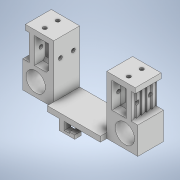
# Autodesk Inventor part: suporte estruzor 1
Saved by Autodesk Inventor 2022 (Build 260153000, 153)
## iProperties
Created: 2022-02-16
Part Number: suporte estruzor 1
Material: Genérico
Document SubType Name: Modeling
Designer: mathe
Density: 1 g/cm^3
Appearance: Padrão
Author: mathe
Autodesk Inventor part; units mm, degrees
ref_plane "YZ Plane" through (0, 0, 0) normal (1, 0, 0) x (0, 1, 0)
ref_plane "XZ Plane" through (0, 0, 0) normal (0, 1, 0) x (-1, 0, 0)
ref_plane "XY Plane" through (0, 0, 0) normal (0, 0, 1) x (1, 0, 0)
sketch "Esboço1" plane through (0, 0, 0) normal (0, 0, 1) x (1, 0, 0)
  line L0 (0, 0) -> (49, 0)
  line L1 (49, 0) -> (49, 41)
  line L2 (0, 41) -> (0, 0)
  line L3 (45, 45) -> (45, 4)
  line L4 (45, 4) -> (4, 4)
  line L5 (4, 4) -> (4, 45)
  line L6 (0, 45) -> (4, 45)
  line L7 (45, 45) -> (49, 45)
  line L8 (45, 45) -> (67, 45)
  line L9 (4, 45) -> (-18, 45)
  line L10 (-18, 45) -> (0, 45)
  line L11 (0, 41) -> (-18, 41)
  line L12 (-18, 41) -> (-18, 45)
  line L13 (67, 45) -> (49, 45)
  line L14 (49, 41) -> (67, 41)
  line L15 (67, 41) -> (67, 45)
  constraints: 32 end point, 5 horizontal, 4 parallel, 2 perpendicular, 1 point on line
extrude "Extrusão1" add sketch "Esboço1" along normal blind 20
sketch "Esboço2" plane through (0, 0, 20) normal (0, 0, 1) x (1, 0, 0)
  line L0 (45, 4) -> (4, 4) projected
  line L1 (0, 0) -> (49, 0) projected
  line L2 (4, 4) -> (45, 4)
  line L3 (45, 4) -> (45, 0)
  line L4 (4, 0) -> (4, 4)
  line L5 (0, 0) -> (49, 0) projected
  line L6 (13.1194, 0) -> (13.1194, -8)
  line L7 (13.1194, -8) -> (23.1194, -8)
  line L8 (23.1194, -8) -> (25.1194, -8)
  line L9 (25.1194, -8) -> (25.1194, -5)
  line L10 (25.1194, -5) -> (21.1194, -5)
  line L11 (21.1194, -5) -> (21.1194, -6)
  line L12 (21.1194, -6) -> (17.1194, -6)
  line L13 (17.1194, -6) -> (17.1194, 0)
  line L14 (45, 0) -> (17.1194, 0)
  line L15 (13.1194, 0) -> (4, 0)
  dimension "d9" = 41
  dimension "d12" = 8
  dimension "d13" = 10
  dimension "d14" = 2
  dimension "d15" = 3
  dimension "d16" = 4
  dimension "d17" = 1
  dimension "d18" = 4
  constraints: 26 end point, 8 perpendicular, 4 point on line, 3 parallel, 1 horizontal
  measures "d9" distance of L3.end L4.start
  measures "d12" distance of L6.start L6.end
  measures "d13" distance of L6.end L7.end
  measures "d14" distance of L7.end L8.end
  measures "d15" distance of L8.end L9.end
  measures "d16" distance of L9.end L10.end
  measures "d17" distance of L10.end L11.end
  measures "d18" distance of L11.end L12.end
extrude "Extrusão2" add sketch "Esboço2" along normal blind 5
sketch "Esboço3" plane through (49, 0, 0) normal (1, 0, 0) x (0, 0, -1)
  line L0 (0, 41) -> (-20, 41) projected
  line L1 (-8.5, 41) -> (-8.5, 21)
  line L2 (-11.5, 41) -> (-11.5, 21)
  line L3 (-11.5, 21) -> (-8.5, 21)
  point P0 (0, 0)
  constraints: 6 end point, 1 horizontal
extrude "Extrusão3" add sketch "Esboço3" along normal blind 15
sketch "Esboço5" plane through (0, 0, 0) normal (-1, 0, 0) x (0, 0, 1)
  line L0 (11.5, 41) -> (11.5, 21) projected
  line L1 (11.5, 41) -> (11.5, 21)
  line L2 (8.5, 21) -> (8.5, 41) projected
  line L3 (11.5, 21) -> (8.5, 21)
  line L4 (8.5, 21) -> (8.5, 41)
  line L5 (8.5, 41) -> (11.5, 41)
  line L6 (0, 41) -> (20, 41) projected
  point P0 (0, 0)
  constraints: 8 end point, 2 collinear, 1 perpendicular, 1 vertical
extrude "Extrusão4" add sketch "Esboço5" along normal blind 15
sketch "Esboço7" plane through (-18, 45, 0) normal (0, 1, 0) x (1, 0, 0)
  line L0 (22, 0) -> (0, 0) projected
  line L1 (22, -20) -> (0, -20) projected
  line L2 (85, -20) -> (63, -20) projected
  line L3 (85, 0) -> (63, 0) projected
  line L4 (0, 0) -> (0, -20) projected
  line L5 (85, 0) -> (85, -20) projected
  point P0 (18, 0)
  point P1 (10, -15)
  point P2 (10, -5)
  point P3 (75, -5)
  point P4 (75, -15)
  dimension "d44" = 5
  dimension "d45" = 5
  dimension "d46" = 5
  dimension "d47" = 5
  dimension "d49" = 10
  dimension "d50" = 10
  dimension "d51" = 10
  dimension "d52" = 10
  measures "d44" distance from line of L0 point (10, -5)
  measures "d45" distance from line of L1 point (10, -15)
  measures "d46" distance from line of L2 point (75, -15)
  measures "d47" distance from line of L3 point (75, -5)
  measures "d49" distance from line of L4 point (10, -15)
  measures "d50" distance from line of L4 point (10, -5)
  measures "d51" distance from line of L5 point (75, -15)
  measures "d52" distance from line of L5 point (75, -5)
hole "Furo1" at (-8, 45, 15) at (-8, 45, 5) at (57, 45, 5) at (57, 45, 15) direction (0, -1, 0) diameter 3 end through all
sketch "Esboço8" plane through (0, 0, 20) normal (0, 0, 1) x (1, 0, 0)
  line L0 (0, 0) -> (4, 0) projected
  line L1 (0, 0) -> (-20, 0)
  line L2 (-20, 0) -> (-20, 21)
  line L3 (-20, 21) -> (0, 21)
  line L4 (0, 21) -> (0, 0)
  line L5 (45, 0) -> (49, 0) projected
  line L6 (49, 0) -> (69, 0)
  line L7 (69, 0) -> (69, 21)
  line L8 (69, 21) -> (49, 21)
  line L9 (49, 21) -> (49, 0)
  circle A0 centre (-10, 10.5) radius 7.5
  circle A1 centre (59, 10.5) radius 7.5
  dimension "d38" = 20
  dimension "d39" = 20
  dimension "d40" = 15
  dimension "d41" = 15
  constraints: 16 end point, 4 parallel, 2 centre point, 2 horizontal, 2 perpendicular
  measures "d38" distance of L2.end L3.end
  measures "d39" distance of L8.end L7.end
  measures "d40" diameter of A0
  measures "d41" diameter of A1
extrude "Extrusão6" add sketch "Esboço8" against normal up to surface (20 mm away)
sketch "Esboço10" plane through (64, 0, 0) normal (1, 0, 0) x (0, 0, -1)
  line L0 (0, 21) -> (-8.5, 21) projected
  line L1 (-20, 45) -> (-20, 4) projected
  line L2 (0, 21) -> (-20, 21)
  line L3 (-20, 21) -> (-20, 41.1382)
  line L4 (-20, 41.1382) -> (0, 41.1382)
  line L5 (0, 41.1382) -> (0, 21)
  point P0 (0, 0)
  point P1 (-6.5, 21)
  point P2 (-6.5, 21)
  constraints: 8 end point, 2 parallel, 1 horizontal, 1 perpendicular, 1 point on line
extrude "Extrusão7" add sketch "Esboço10" against normal blind 4
sketch "Esboço12" plane through (-15, 0, 0) normal (-1, 0, 0) x (0, 0, 1)
  line L0 (0, 21) -> (20, 21) projected
  line L1 (0, 41) -> (8.5, 41) projected
  line L2 (20, 21) -> (0, 21)
  line L3 (0, 21) -> (0, 41)
  line L4 (0, 41) -> (20, 41)
  line L5 (20, 41) -> (20, 21)
  point P0 (0, 0)
  point P1 (13.5, 21)
  point P2 (6.5, 41)
  point P3 (13.5, 21)
  point P4 (6.5, 41)
  constraints: 8 end point, 2 parallel, 1 horizontal, 1 perpendicular
extrude "Extrusão8" add sketch "Esboço12" against normal blind 4
sketch "Esboço15" plane through (64, 0, 0) normal (1, 0, 0) x (0, 0, -1)
  point P0 (0, 0)
  point P1 (-5, 31)
  point P2 (-15, 31)
hole "Furo2" at (64, 31, 5) at (64, 31, 15) direction (-1, 0, 0) diameter 3 end through all
sketch "Esboço13" plane through (-20, 21, 20) normal (0, 1, 0) x (1, 0, 0)
  line L0 (5, 0) -> (6.0353, 3.8637)
  line L1 (5, 0) -> (9, 0) construction
  line L2 (6.0353, 3.8637) -> (5, 4.1411)
  line L3 (5, 0) -> (5, 20) projected
  line L4 (5, 4) -> (6.0353, 7.8637)
  line L5 (6.0353, 7.8637) -> (5, 8.1411)
  line L6 (5, 8) -> (6.0353, 11.8637)
  line L7 (6.0353, 11.8637) -> (5, 12.1411)
  line L8 (5, 12) -> (6.0353, 15.8637)
  line L9 (6.0353, 15.8637) -> (5, 16.1411)
  line L10 (5, 16) -> (6.0353, 19.8637)
  line L11 (6.0353, 19.8637) -> (5, 20.1411)
  line L12 (5, 20) -> (6.0353, 23.8637)
  line L13 (6.0353, 23.8637) -> (5, 24.1411)
  line L14 (5, 24) -> (6.0353, 27.8637)
  line L15 (6.0353, 27.8637) -> (5, 28.1411)
  line L16 (5, 28) -> (6.0353, 31.8637)
  line L17 (6.0353, 31.8637) -> (5, 32.1411)
  line L18 (5, 32) -> (6.0353, 35.8637)
  line L19 (6.0353, 35.8637) -> (5, 36.1411)
  line L20 (5, 36) -> (6.0353, 39.8637)
  line L21 (6.0353, 39.8637) -> (5, 40.1411)
  line L22 (5, 0) -> (4.0983, 0)
  line L23 (5, 0) -> (0, 0) projected
  line L24 (4.0983, 0) -> (4.5493, 24.0085)
  line L25 (4.5493, 24.0085) -> (5, 24)
  line L26 (33.1194, 0) -> (45.1194, 0) projected
  line L27 (44.5, 0) -> (44.5, 16.8251)
  line L28 (84, 0) -> (82.9647, 3.8637)
  line L29 (84, 0) -> (80, 0) construction
  line L30 (82.9647, 3.8637) -> (84, 4.1411)
  line L31 (84, 4) -> (82.9647, 7.8637)
  line L32 (82.9647, 7.8637) -> (84, 8.1411)
  line L33 (84, 8) -> (82.9647, 11.8637)
  line L34 (82.9647, 11.8637) -> (84, 12.1411)
  line L35 (84, 12) -> (82.9647, 15.8637)
  line L36 (82.9647, 15.8637) -> (84, 16.1411)
  line L37 (84, 16) -> (82.9647, 19.8637)
  line L38 (82.9647, 19.8637) -> (84, 20.1411)
  line L39 (84, 20) -> (82.9647, 23.8637)
  line L40 (82.9647, 23.8637) -> (84, 24.1411)
  line L41 (84, 24) -> (82.9647, 27.8637)
  line L42 (82.9647, 27.8637) -> (84, 28.1411)
  line L43 (84, 28) -> (82.9647, 31.8637)
  line L44 (82.9647, 31.8637) -> (84, 32.1411)
  line L45 (84, 32) -> (82.9647, 35.8637)
  line L46 (82.9647, 35.8637) -> (84, 36.1411)
  line L47 (84, 36) -> (82.9647, 39.8637)
  line L48 (82.9647, 39.8637) -> (84, 40.1411)
  line L49 (84, 0) -> (84.9017, 0)
  line L50 (84, 0) -> (89, 0)
  line L51 (84.9017, 0) -> (84.4507, 24.0085)
  line L52 (84.4507, 24.0085) -> (84, 24)
  point P0 (20, 20)
  point P1 (69, 20)
  point P2 (83.9647, 24.1317)
  point P3 (83.9647, 20.1317)
  point P4 (83.9647, 16.1317)
  point P5 (83.9647, 12.1317)
  point P6 (83.9647, 8.1317)
  point P7 (83.9647, 4.1317)
  point P8 (5.0353, 4.1317)
  point P9 (5, 4)
  point P10 (5.0353, 8.1317)
  point P11 (5.0353, 12.1317)
  point P12 (5.0353, 16.1317)
  point P13 (5.0353, 20.1317)
  point P14 (5.0353, 24.1317)
  dimension "d60" = 4
  dimension "d61" = 75
  dimension "d64" = 4
  constraints: 100 end point, 35 symmetric about line, 4 point on line, 2 perpendicular, 2 vertical, 1 equal length, 1 horizontal, 45 other
  measures "d60" distance of L0.start L0.end
  measures "d61" angle of L1 L0
  measures "d64" distance of L0.end L4.end
extrude "Extrusão10" cut sketch "Esboço13" along normal up to surface (20 mm away) contours L3 L4 L2 L0 | L22 L24 L25 L14 L13 L12 L3 | L2 L3 L6 L5 L4 | L5 L3 L8 L7 L6 | L7 L3 L10 L9 L8 | L11 L10 L9 L3 L12 | L28 L30 L31 L32 L33 L34 L35 L36 L37 L38 L39 L40 L41 L52 L51 L49
chamfer "Chanfro3" distance 2 angle 45 8 edges at (49, 31, 8.5) (54.5, 21, 8.5) (49, 31, 11.5) (54.5, 21, 11.5) (-5.5, 21, 11.5) (0, 21, 15.75) (0, 31, 8.5) (-5.5, 21, 8.5)
